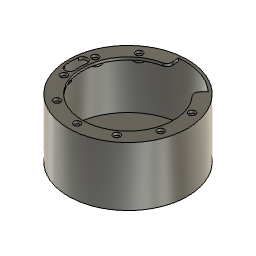
CoozieAssm (Autodesk Fusion 360 archive; units mm, degrees)
design "BatteryPack"
Autodesk Fusion 360 part; units mm, degrees
sketch "Sketch1" plane through (0, 0, 0) normal (0, 0, 1) x (1, 0, 0)
  circle A0 centre (0, 0) radius 44.5
  circle A1 centre (0, 0) radius 42.5
  dimension "d1" = 89
  dimension "d2" = 2
  constraint coincident A0.centre A1.centre
  measures "d1" diameter of A0
  measures "d2" distance of A0 A1
extrude "Extrude1" add sketch "Sketch1" against normal blind 2 contours A0 | A1 makes body 1
extrude "Extrude2" add sketch "Sketch1" along normal blind 40 bodies 1
sketch "Sketch2" plane through (0, 0, 40) normal (0, 0, 1) x (-1, 0, 0)
  circle A0 centre (0, 0) radius 42.5
  circle A1 centre (0, 0) radius 44.5
  circle A2 centre (0, 0) radius 44.5
  dimension "d7" = 89
  constraint concentric A0 A2
  measures "d7" diameter of A2
extrude "Extrude3" add sketch "Sketch2" along normal blind 2 separate body contours A0 | A1 A2 makes body 2
sketch "Sketch3" plane through (0, 0, 42) normal (0, 0, 1) x (-1, 0, 0)
  circle A0 centre (0, 0) radius 44.5
  circle A1 centre (0, -38) radius 2.5
  circle A2 centre (0, -38) radius 4
  dimension "d10" = 5
  dimension "d12" = 1.5
  dimension "d24" = 38
  constraint concentric A1 A2
  constraint vertical A0.centre A1.centre
  measures "d10" diameter of A1
  measures "d12" distance of A1 A2
  measures "d24" distance of A0.centre A1.centre
extrude "Extrude4" add sketch "Sketch3" against normal blind 3.5 contours A1 | A2 bodies 2
extrude "Extrude5" cut sketch "Sketch3" against normal blind 2 contours A1 bodies 2
pattern_circular "C-Pattern1" count 10 over 360 about axis through (0, 0, 1.75) along (0, 0, 1) of "Extrude4", "Extrude5"
sketch "Sketch5" plane through (0, 0, 42) normal (0, 0, 1) x (-1, 0, 0)
  circle A0 centre (0, 38) radius 2.5
  circle A1 centre (22.3358, 30.7426) radius 2.5
  circle A2 centre (36.1401, 11.7426) radius 2.5
  circle A3 centre (36.1401, -11.7426) radius 2.5
  circle A4 centre (22.3358, -30.7426) radius 2.5
  circle A5 centre (0, -38) radius 2.5
  circle A6 centre (0, 0) radius 44.5
  circle A7 centre (0, 0) radius 34
  circle A8 centre (0, -38) radius 4
  circle A9 centre (-36.1401, -11.7426) radius 2.5
  circle A10 centre (-36.1401, 11.7426) radius 2.5
  circle A11 centre (-22.3358, 30.7426) radius 2.5
  circle A12 centre (-22.3358, -30.7426) radius 2.5
  constraint concentric A6 A7
  constraint tangent A7 A8
extrude "Extrude6" cut sketch "Sketch5" against normal blind 5 contours A7 bodies 2
sketch "Sketch7" plane through (0, 0, 42) normal (0, 0, 1) x (-1, 0, 0)
  circle A0 centre (0, 0) radius 34
  circle A1 centre (0, 38) radius 2.5
  circle A2 centre (22.3358, 30.7426) radius 2.5
  circle A3 centre (36.1401, 11.7426) radius 2.5
  circle A4 centre (36.1401, -11.7426) radius 2.5
  circle A5 centre (22.3358, -30.7426) radius 2.5
  circle A6 centre (0, -38) radius 2.5
  circle A7 centre (0, 0) radius 44.5
  arc A8 (42.1904, -5.1205) -> (42.1904, 5.1205) centre (0, 0) ccw
  arc A9 (35.2414, -4.2771) -> (42.1904, -5.1205) centre (38.7159, -4.6988) ccw
  arc A10 (35.2414, -4.2771) -> (35.2414, 4.2771) centre (0, 0) ccw
  arc A11 (42.1904, 5.1205) -> (35.2414, 4.2771) centre (38.7159, 4.6988) ccw
  arc A12 (38.7159, -4.6988) -> (38.7159, 4.6988) centre (0, 0) ccw construction
  circle A13 centre (-36.1401, -11.7426) radius 2.5
  circle A14 centre (-36.1401, 11.7426) radius 2.5
  circle A15 centre (-22.3358, 30.7426) radius 2.5
  circle A16 centre (-22.3358, -30.7426) radius 2.5
  circle A17 centre (36.1401, -11.7426) radius 4
  circle A18 centre (36.1401, 11.7426) radius 4
  dimension "d25" = 2
  dimension "d26" = 39
  constraint tangent A8 A9
  constraint tangent A9 A10
  constraint tangent A10 A11
  constraint tangent A8 A11
  constraint coincident A0.centre A7.centre
  constraint tangent A9 A17
  constraint tangent A11 A18
  measures "d25" distance of A7 A8
  measures "d26" radius of A12
extrude "Extrude7" cut sketch "Sketch7" against normal blind 5 contours A8 A9 A10 A11 bodies 2
combine "Combine1" operation add target body 1 tool bodies 2
sketch "Sketch9" plane through (0, 0, 42) normal (0, 0, 1) x (-1, 0, 0)
  circle A0 centre (0, 0) radius 44.5 construction
  line L0 (0, 0) -> (4.6842, -44.2528)
  line L1 (0, 0) -> (-29.8007, -33.0479)
  circle A1 centre (0, 0) radius 34 construction
  circle A2 centre (0, 0) radius 42.5
  circle A3 centre (22.3358, 30.7426) radius 4
  circle A4 centre (0, 38) radius 4
  constraint coincident A0.centre L0.start
  constraint coincident A0 L0.end
  constraint coincident A0 L1.end
  constraint tangent L1 A3
  constraint tangent L0 A4
extrude "Extrude8" cut sketch "Sketch9" against normal blind 6 contours L0 L1 A2 picked at (1.0038, -28.2462) bodies 1
fillet "Fillet1" radius 4 2 edges at (-3.5789, 33.8111, 41) (22.7691, 25.2501, 41) on bodies 1
